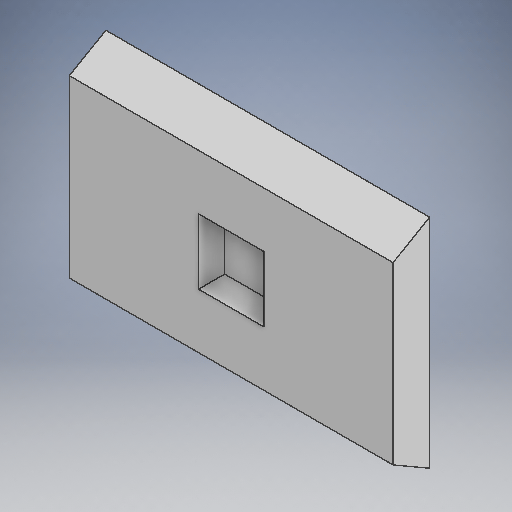
# Autodesk Inventor part: door
Saved by Autodesk Inventor 2025.2 (Build 292293000, 293)
## iProperties
Created: 2025-03-09
Part Number: door
Material: Generic
Document SubType Name: Modeling
Designer: Alex
Density: 1 g/cm^3
Appearance: Default
Author: Alex
Autodesk Inventor part; units mm, degrees
ref_plane "YZ Plane" through (0, 0, 0) normal (1, 0, 0) x (0, 1, 0)
sketch "Sketch1" plane through (0, 0, 0) normal (1, 0, 0) x (0, 1, 0)
  line L0 (0, 0) -> (1.7321, 3) construction
  line L1 (1.7321, 3) -> (15.2679, 3) construction
  line L2 (15.2679, 3) -> (17, 0) construction
  line L3 (17, 0) -> (0, 0) construction
  line L4 (15.2679, 3) -> (15.2679, 0) construction
  line L5 (0.1732, 0.1) -> (1.7898, 2.9)
  line L6 (1.7898, 2.9) -> (15.2102, 2.9)
  line L7 (15.2102, 2.9) -> (16.8268, 0.1)
  line L8 (16.8268, 0.1) -> (0.1732, 0.1)
  line L9 (16.0185, 1.5) -> (16.1051, 1.55) construction
  dimension "d0" = 60
  dimension "d1" = 17
  dimension "d2" = 3
  dimension "d11" = 0.1
  constraints: 20 end point, 2 parallel, 2 perpendicular, 2 point on line, 1 equal length, 1 horizontal, 1 midpoint, 3 other
  measures "d0" angle of L3 L0
  measures "d1" distance of L0.start L2.end
  measures "d2" distance of L1.end L4.end
  measures "d11" distance between parallel lines of L3 L8
extrude "Extrusion1" add sketch "Sketch1" along normal blind 24.8
sketch "Sketch3" plane through (0, 1.7898, 2.9) normal (0, 0, 1) x (1, 0, 0)
  line L0 (0, 13.4204) -> (0, 0) construction
  line L1 (0, 13.4204) -> (24.8, 13.4204) construction
  line L2 (0, 0) -> (3, 0) construction
  line L3 (3, 0) -> (3, 13.4204) construction
  line L4 (3, 13.4204) -> (0, 13.4204) construction
  line L5 (0, 13.4204) -> (0, 0) construction
  circle A0 centre (1.5, 6.7102) radius 1.0891
  line L6 (0, 6.7102) -> (3, 6.7102) construction
  point P0 (0, -1.7898)
  point P1 (1.5, 13.4204)
  dimension "d12" = 3
  constraints: 10 end point, 3 midpoint, 2 parallel, 1 centre point, 1 horizontal, 1 horizontal alignment, 1 perpendicular, 1 point on line, 1 vertical alignment
  measures "d12" distance between parallel lines of L3 L0
ref_plane "Work Plane1" through (1.5, 8.5, 2.9) normal (1, 0, 0) x (0, 1, 0)
sketch "Sketch5" plane through (0, 0.1732, 0.1) normal (0, 0, -1) x (-1, 0, 0)
  line L0 (0, 0) -> (0, 16.6536) construction
  line L1 (0, 16.6536) -> (-24.8, 16.6536) construction
  line L2 (-24.8, 0) -> (-24.8, 16.6536) construction
  line L3 (0, 0) -> (-24.8, 0) construction
  line L4 (-21.8, 0) -> (-21.8, 16.6536) construction
  line L5 (-24.8, 8.3268) -> (-21.8, 8.3268) construction
  point P0 (0, -0.1732)
  point P1 (-23.3, 8.3268)
  dimension "d16" = 3
  constraints: 4 end point, 3 midpoint, 2 point on line, 1 parallel
  measures "d16" distance between parallel lines of L4 L2
ref_plane "Work Plane2" through (23.3, 8.5, 0.1) normal (-1, 0, 0) x (0, -1, 0)
sketch "Sketch6" plane through (23.3, 8.5, 0.1) normal (-1, 0, 0) x (0, -1, 0)
  line L0 (8.3268, 0) -> (-8.3268, 0) projected
  line L1 (0, 0) -> (0, -1)
  line L2 (0, 0) -> (-1, 0)
  arc A0 (-1, 0) -> (0, -1) centre (0, 0) ccw
  point P0 (8.5, -0.1)
  dimension "d17" = 1
  constraints: 4 end point, 2 line through centre, 2 point on circle, 1 centre point, 1 midpoint, 1 point on line, 1 vertical
  measures "d17" distance of L1.start L1.end
revolve "Revolution2" add sketch "Sketch6" angle 360 about axis through (23.3, 8.5, 0.1) along (0, 0, -1)
fillet "Fillet4" radius 0.3 1 edges at (23.3, 7.5, 0.1)
sketch "Sketch7" plane through (0, 1.7898, 2.9) normal (0, 0, 1) x (1, 0, 0)
  line L0 (9.9, 4.2102) -> (14.9, 4.2102)
  line L1 (14.9, 4.2102) -> (14.9, 9.2102)
  line L2 (14.9, 9.2102) -> (9.9, 9.2102)
  line L3 (9.9, 9.2102) -> (9.9, 4.2102)
  line L4 (0, 13.4204) -> (0, 0) projected
  line L5 (0, 13.4204) -> (24.8, 13.4204) projected
  point P0 (0, -1.7898)
  point P1 (9.9, 6.7102)
  point P2 (0, 6.7102)
  point P3 (12.4, 9.2102)
  point P4 (12.4, 13.4204)
  dimension "d20" = 5
  dimension "d21" = 5
  constraints: 8 end point, 4 midpoint, 2 parallel, 1 horizontal, 1 horizontal alignment, 1 perpendicular, 1 vertical alignment
  measures "d20" distance of L1.end L2.end
  measures "d21" distance of L2.end L0.start
extrude "Extrusion3" cut sketch "Sketch7" against normal blind 1
fillet "Fillet5" radius 1 4 edges at (9.9, 8.5, 1.9) (12.4, 6, 1.9) (14.9, 8.5, 1.9) (12.4, 11, 1.9)
body "Solid1"
